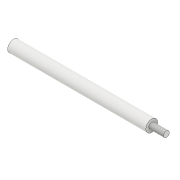
# Autodesk Inventor part: brazos_planetarios1
Saved by Autodesk Inventor 2022 (Build 260153000, 153)
## iProperties
Created: 2019-06-24
Part Number: brazos_planetarios1
Material: Acetal Resin, Black
Document SubType Name: Modeling
Designer: Cristiano
Density: 1.425 g/cm^3
Appearance: Blanco
Author: Cristiano
Autodesk Inventor part; units mm, degrees
ref_plane "YZ Plane" through (0, 0, 0) normal (1, 0, 0) x (0, 1, 0)
ref_plane "XZ Plane" through (0, 0, 0) normal (0, 1, 0) x (-1, 0, 0)
sketch "Boceto1" plane through (0, 0, 0) normal (0, 1, 0) x (-1, 0, 0)
  line L0 (0, 0) -> (235, 0)
  line L1 (235, 0) -> (235, -10)
  line L2 (235, -20) -> (0, -20) construction
  line L3 (0, -20) -> (0, -10) construction
  line L4 (235, -10) -> (0, -10)
  line L5 (235, -10) -> (235, -20) construction
  line L6 (0, -10) -> (0, 0)
  dimension "d0" = 20
  dimension "d1" = 235
  constraints: 14 end point, 5 parallel, 2 perpendicular, 1 horizontal
  measures "d0" distance of L2.end L0.start
  measures "d1" distance of L0.start L0.end
ref_plane "Plano de trabajo2" through (0, 0, 0) normal (1, 0, 0) x (0, 0, -1)
revolve "Revolución1" add sketch "Boceto1" angle 360 about axis through (-235, 0, -10) along (1, 0, 0)
sketch "Boceto4" plane through (0, 0, 0) normal (1, 0, 0) x (0, 0, -1)
  circle A0 centre (10, 0) radius 5
  circle A1 centre (10, 0) radius 10 construction
  point P0 (0, 0)
  dimension "d23" = 10
  constraints: 1 centre point, 1 horizontal alignment, 1 other
  measures "d23" diameter of A0
extrude "Extrusión5" add sketch "Boceto4" along normal blind 25
thread "Rosca4" size "M10x1.5" class "6g" standard "ANSI Metric M Profile" full length
